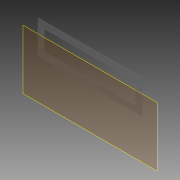
# Autodesk Inventor part: ReflectiveImage01
Saved by Autodesk Inventor 2013 (Build 170138000, 138)
## iProperties
Created: 2013-01-04
Part Number: ReflectiveImage01
Material: Polycarbonate, Clear
Document SubType Name: Modeling
Designer: Phillip
Density: 1 g/cm^3
Author: Phillip
Autodesk Inventor part; units mm, degrees
ref_plane "YZ Plane" through (0, 0, 0) normal (1, 0, 0) x (0, 1, 0)
ref_plane "XZ Plane" through (0, 0, 0) normal (0, 1, 0) x (-1, 0, 0)
ref_plane "XY Plane" through (0, 0, 0) normal (0, 0, 1) x (1, 0, 0)
ref_plane "Work Plane1" through (0, 0, 0) normal (0, 0, 1) x (1, 0, 0)
sketch "Sketch1" plane through (0, 0, 0) normal (0, 0, 1) x (1, 0, 0)
  line L0 (685.8, 273.3086) -> (-685.8, 273.3086) projected
  line L1 (685.8, 425.7086) -> (685.8, 273.3086) projected
  line L2 (685.8, 578.1086) -> (685.8, 425.7086) projected
  line L3 (-685.8, 578.1086) -> (685.8, 578.1086) projected
  line L4 (-685.8, 425.7086) -> (-685.8, 578.1086) projected
  line L5 (-685.8, 273.3086) -> (-685.8, 425.7086) projected
  line L6 (685.8, 578.1086) -> (-685.8, 578.1086)
  line L7 (-685.8, 578.1086) -> (-685.8, 273.3086)
  line L8 (-685.8, 273.3086) -> (685.8, 273.3086)
  line L9 (685.8, 273.3086) -> (685.8, 578.1086)
  line L10 (787.4, 171.7086) -> (-787.4, 171.7086)
  line L11 (-787.4, 171.7086) -> (-787.4, 679.7086)
  line L12 (-787.4, 679.7086) -> (787.4, 679.7086)
  line L13 (787.4, 679.7086) -> (787.4, 171.7086)
  point P0 (0, 0)
  dimension "d0" = 101.6
  constraints: 16 end point, 4 parallel, 2 perpendicular, 1 horizontal, 3 other
  measures "d0" distance between parallel lines of L0 L10
extrude "Extrusion1" add sketch "Sketch1" along normal blind 2.54
body "Solid1"
